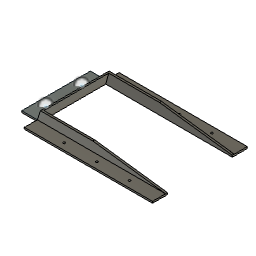
Fender Vent v8 (Autodesk Fusion 360 design; units mm, degrees)
Autodesk Fusion 360 part; units mm, degrees
sketch "Sketch1" plane through (0, 0, 0) normal (0, 0, 1) x (1, 0, 0)
  line L0 (0, 0) -> (200, 0)
  line L1 (200, 0) -> (200, 105)
  line L2 (200, 105) -> (0, 105)
  line L3 (0, 105) -> (0, 0)
  line L4 (0, 105) -> (200, 105)
  line L5 (0, -20) -> (-20, -20)
  line L6 (-20, -20) -> (-20, 125)
  line L7 (-20, 125) -> (0, 125)
  line L8 (0, 125) -> (0, -20)
  line L9 (0, 105) -> (200, 105)
  line L10 (200, 105) -> (200, 125)
  line L11 (200, 125) -> (0, 125)
  line L12 (0, 125) -> (0, 105)
  line L13 (0, 0) -> (200, 0)
  line L14 (200, 0) -> (200, -20)
  line L15 (200, -20) -> (0, -20)
  line L16 (0, -20) -> (0, 0)
  line L17 (0, 105) -> (200, 105)
  line L18 (200, 105) -> (200, 102)
  line L19 (200, 102) -> (0, 102)
  line L20 (0, 102) -> (0, 105)
  line L21 (0, 0) -> (200, 0)
  line L22 (200, 0) -> (200, 3)
  line L23 (200, 3) -> (0, 3)
  line L24 (0, 3) -> (0, 0)
  line L25 (0, 102) -> (4, 102)
  line L26 (4, 102) -> (4, 3)
  line L27 (4, 3) -> (0, 3)
  line L28 (0, 3) -> (0, 102)
  dimension "d1" = 200
  dimension "d2" = 105
  dimension "d7" = 20
  dimension "d8" = 145
  dimension "d9" = 200
  dimension "d10" = 20
  dimension "d11" = 200
  dimension "d12" = 20
  dimension "d13" = 3
  dimension "d14" = 200
  dimension "d15" = 3
  dimension "d16" = 4
  constraint horizontal L0
  constraint vertical L1
  constraint horizontal L2
  constraint vertical L3
  constraint coincident L0.start L3.end
  constraint horizontal L4
  constraint horizontal L5
  constraint vertical L6
  constraint horizontal L7
  constraint vertical L8
  constraint horizontal L9
  constraint vertical L10
  constraint horizontal L11
  constraint vertical L12
  constraint horizontal L13
  constraint vertical L14
  constraint horizontal L15
  constraint vertical L16
  constraint horizontal L17
  constraint vertical L18
  constraint horizontal L19
  constraint vertical L20
  constraint horizontal L21
  constraint vertical L22
  constraint horizontal L23
  constraint vertical L24
  constraint horizontal L25
  constraint vertical L26
  constraint horizontal L27
  constraint vertical L28
  measures "d1" distance of L0.start L0.end
  measures "d2" distance of L0.start L2.end
  measures "d7" distance of L5.start L5.end
  measures "d8" distance of L5.start L7.end
  measures "d9" distance of L2.end L1.end
  measures "d10" distance of L2.end L7.end
  measures "d11" distance of L0.start L0.end
  measures "d12" distance of L0.start L5.start
  measures "d13" distance of L2.end L19.end
  measures "d14" distance of L0.start L0.end
  measures "d15" distance of L0.start L23.end
  measures "d16" distance of L19.end L25.end
extrude "Extrude1" add sketch "Sketch1" along normal blind 5 contours L0 L1 L3 L8 L13 L21 L22 L23 L24 L27 | L3 L5 L6 L7 L8 L12 L16 L20 L24 L28 | L0 L8 L13 L14 L15 L16 L21 | L1 L2 L3 L4 L8 L9 L17 L18 L19 L20 L25 | L2 L4 L8 L9 L10 L11 L12 L17 makes body 1
extrude "Extrude2" add sketch "Sketch1" along normal blind 20 separate body contours L3 L8 L19 L23 L25 L26 L27 L28 makes body 2
sketch "Sketch3" plane through (0, 0, 0) normal (0, 1, 0) x (1, 0, 0)
  line L0 (0, -25) -> (85, -25)
  line L1 (85, -25) -> (85, -5)
  line L2 (85, -5) -> (0, -5)
  line L3 (0, -5) -> (0, -25)
  line L4 (85, -25) -> (200, -5)
  line L5 (200, -5) -> (85, -5)
  constraint horizontal L0
  constraint vertical L1
  constraint horizontal L2
  constraint vertical L3
  constraint perpendicular L1 L5
extrude "Extrude3" add sketch "Sketch3" along normal blind 3 bodies 1 2
extrude "Extrude4" add sketch "Sketch1" along normal blind 25 separate body contours L3 L8 L19 L23 L25 L26 L27 L28 makes body 3
sketch "Sketch5" plane through (0, 102, 0) normal (0, 1, 0) x (-1, 0, 0)
  line L0 (-4, 0) -> (0, 0)
  line L1 (0, 0) -> (0, 25)
  line L2 (0, 25) -> (-4, 25)
  line L3 (-4, 25) -> (-4, 0)
  line L4 (-4, 25) -> (-85, 25)
  line L5 (-85, 25) -> (-85, 5)
  line L6 (-85, 5) -> (-4, 5)
  line L7 (-4, 5) -> (-4, 25)
  line L8 (-85, 25) -> (-200, 5)
  line L9 (-200, 5) -> (-85, 5)
  constraint horizontal L4
  constraint vertical L5
  constraint horizontal L6
  constraint vertical L7
  constraint coincident L2.end L3.start
  constraint perpendicular L5 L9
extrude "Extrude5" add sketch "Sketch5" along normal blind 3 separate body contours L3 L4 L5 L6 L7 | L5 L8 L9 makes body 4
extrude "Extrude6" add 1 faces at (4, 103, 18.3333) along direction (-1, 0, 0) blind 4 on bodies 4 bodies 1 4 3
extrude "Extrude7" cut sketch "Sketch1" along normal blind 1 contours L0 L1 L3 L8 L13 L21 L22 L23 L24 L27 | L3 L5 L6 L7 L8 L12 L16 L20 L24 L28 | L0 L8 L13 L14 L15 L16 L21 | L3 L8 L19 L23 L25 L26 L27 L28 | L1 L2 L3 L4 L8 L9 L17 L18 L19 L20 L25 | L2 L4 L8 L9 L10 L11 L12 L17 bodies 1
extrude "Extrude8" cut 1 faces at (-12, 36, 1) along direction (0, 0, 1) blind 1 on bodies 1 bodies 1
extrude "Extrude9" cut 1 faces at (-12, 36, 2) along direction (0, 0, 1) blind 0.5 on bodies 1 bodies 1
delete_face "DeleteFace1" 1 faces at (1.3333, 36, 25) on bodies 1
delete_face "DeleteFace2" 3 faces at (66.6667, 0, 16.5942) (1.3333, 69, 39.5507) (0, 70, 16.5942) on bodies 1
sketch "Sketch6" plane through (0, 0, 0) normal (0, 1, 0) x (1, 0, 0)
  line L0 (4, -5) -> (8.5106, -19.3058)
  line L1 (4, -5) -> (19, -5) construction
  line L2 (8.5106, -19.3058) -> (88.5106, -19.3058)
  line L3 (88.5106, -19.3058) -> (200, -5)
  line L4 (200, -5) -> (4, -5)
  dimension "d33" = 15
  dimension "d34" = 72.5
  dimension "d35" = 80
  constraint horizontal L1
  constraint horizontal L2
  measures "d33" distance of L0.start L0.end
  measures "d34" angle of L0 L1
  measures "d35" distance of L0.end L2.end
extrude "Extrude10" add sketch "Sketch6" along normal blind 3 bodies 1
ref_plane "WorkPlane1" through (102, 102, 10.9029) normal (0, 1, 0) x (-1, 0, 0)
sketch "Sketch9" plane through (0, 102, 0) normal (0, 1, 0) x (1, 0, 0)
  line L0 (4, -5) -> (8.5106, -19.3058)
  line L1 (4, -5) -> (19, -5) construction
  line L2 (8.5106, -19.3058) -> (88.5106, -19.3058)
  line L3 (88.5106, -19.3058) -> (200, -5)
  line L4 (200, -5) -> (4, -5)
  dimension "d39" = 72.5
  dimension "d40" = 15
  dimension "d41" = 80
  constraint horizontal L1
  constraint horizontal L2
  measures "d39" angle of L0 L1
  measures "d40" distance of L0.start L0.end
  measures "d41" distance of L0.end L2.end
extrude "Extrude11" add sketch "Sketch9" along normal blind 3 bodies 1
sketch "Sketch11" plane through (0, 3, 0) normal (0, 1, 0) x (-1, 0, 0)
  line L0 (-200, 5) -> (-200, 2.5)
  line L1 (-200, 2.5) -> (-4, 2.5)
  line L2 (-4, 2.5) -> (-4, 5)
  line L3 (-4, 5) -> (-8.5106, 19.3058)
  line L4 (-8.5106, 19.3058) -> (-88.5106, 19.3058)
  line L5 (-88.5106, 19.3058) -> (-200, 5)
  line L6 (-8.5106, 19.3058) -> (-4, 5)
  line L7 (-4, 2.5) -> (-4, 5)
  line L8 (-4, 2.5) -> (-6.5, 2.5)
  line L9 (-8.5106, 19.3058) -> (-11.0106, 19.3058)
  line L10 (-11.0106, 19.3058) -> (-6.5, 2.5)
  dimension "d44" = 2.5
  dimension "d45" = 2.5
  constraint coincident L3.end L4.start
  constraint coincident L2.end L3.start
  constraint coincident L1.end L2.start
  constraint perpendicular L2 L8
  constraint parallel L4 L9
  measures "d44" distance of L1.end L8.end
  measures "d45" distance of L3.end L9.end
extrude "Extrude12" add sketch "Sketch11" along normal blind 99 contours L1 L2 L3 L4 L6 L7 L8 L9 L10 bodies 1
sketch "Sketch12" plane through (0, 0, 5) normal (0, 0, 1) x (-1, 0, 0)
  line L0 (-4, -105) -> (-200, -105)
  line L1 (-200, -105) -> (-200, -125)
  line L2 (-200, -125) -> (20, -125)
  line L3 (20, -125) -> (20, 20)
  line L4 (20, 20) -> (-200, 20)
  line L5 (-200, 20) -> (-200, 0)
  line L6 (-200, 0) -> (-4, 0)
  line L7 (-4, 0) -> (-4, -3)
  line L8 (-4, -3) -> (-4, -102)
  line L9 (-4, -102) -> (-4, -105)
  line L10 (-4, 0) -> (20, 0)
  line L11 (20, 0) -> (20, 20)
  line L12 (20, 20) -> (-4, 20)
  line L13 (-4, 20) -> (-4, 0)
  constraint horizontal L10
  constraint vertical L11
  constraint horizontal L12
  constraint vertical L13
  constraint coincident L3.end L4.start
  constraint coincident L6.end L7.start
extrude "Extrude13" cut sketch "Sketch12" against normal blind 2.5 contours L3 L4 L10 L11 L12 L13 bodies 1
sketch "Sketch13" plane through (0, 0, 5) normal (0, 0, 1) x (-1, 0, 0)
  line L0 (20, 0) -> (-4, 0)
  line L1 (-4, 0) -> (-4, -3)
  line L2 (-4, -3) -> (-4, -102)
  line L3 (-4, -102) -> (-4, -105)
  line L4 (-4, -105) -> (-200, -105)
  line L5 (-200, -105) -> (-200, -125)
  line L6 (-200, -125) -> (20, -125)
  line L7 (20, -125) -> (20, 0)
  line L8 (-4, -105) -> (20, -105)
  line L9 (20, -105) -> (20, -125)
  line L10 (20, -125) -> (-4, -125)
  line L11 (-4, -125) -> (-4, -105)
  constraint horizontal L8
  constraint vertical L9
  constraint horizontal L10
  constraint vertical L11
  constraint coincident L6.end L7.start
  constraint coincident L3.end L4.start
extrude "Extrude14" cut sketch "Sketch13" against normal blind 2.5 contours L6 L7 L8 L9 L10 L11 bodies 1
move_body "Move1" bodies 1 to x (1, 0, 0) y (0, 1, 0) z (0, 0, 1) at (0, 0, -2.5)
sketch "Sketch14" plane through (0, 0, 2.5) normal (0, 0, 1) x (-1, 0, 0)
  line L0 (-4, -105) -> (20, -105)
  line L1 (20, -105) -> (20, 0)
  line L2 (20, 0) -> (-4, 0)
  line L3 (-4, 0) -> (-4, -3)
  line L4 (-4, -3) -> (-4, -102)
  line L5 (-4, -102) -> (-4, -105)
  circle A0 centre (8, -80) radius 1.6
  circle A1 centre (8, -25) radius 1.6
  dimension "d52" = 3.2
  dimension "d53" = 3.2
  constraint vertical A0.centre A1.centre
  measures "d52" diameter of A0
  measures "d53" diameter of A1
extrude "Extrude15" cut sketch "Sketch14" against normal blind 2.5 contours A0 bodies 1
extrude "Extrude16" cut sketch "Sketch14" against normal blind 2.5 contours A1 bodies 1
sketch "Sketch15" plane through (0, 0, 2.5) normal (0, 0, 1) x (-1, 0, 0)
  line L0 (-4, -125) -> (-4, -105)
  line L1 (-4, -105) -> (-200, -105)
  line L2 (-200, -105) -> (-200, -125)
  line L3 (-200, -125) -> (-4, -125)
  circle A0 centre (-55, -115.8072) radius 1.6
  circle A1 centre (-105, -115.8072) radius 1.6
  circle A2 centre (-55, 10) radius 1.6
  circle A3 centre (-105, 10) radius 1.6
  circle A4 centre (-155, -115.8072) radius 1.6
  circle A5 centre (-155, 10) radius 1.6
  dimension "d58" = 3.2
  dimension "d59" = 3.2
  dimension "d60" = 3.2
  dimension "d61" = 3.2
  dimension "d62" = 3.2
  dimension "d63" = 3.2
  constraint vertical A1.centre A3.centre
  constraint vertical A0.centre A2.centre
  constraint horizontal A0.centre A1.centre
  constraint horizontal A2.centre A3.centre
  constraint horizontal A3.centre A5.centre
  constraint horizontal A1.centre A4.centre
  constraint vertical A4.centre A5.centre
  measures "d58" diameter of A0
  measures "d59" diameter of A1
  measures "d60" diameter of A2
  measures "d61" diameter of A3
  measures "d62" diameter of A4
  measures "d63" diameter of A5
extrude "Extrude17" cut sketch "Sketch15" against normal blind 2.5 contours A0 | A1 | A2 | A3 | A4 | A5 bodies 1
